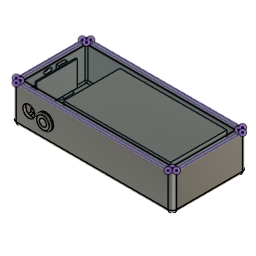
battery_box v25 (Autodesk Fusion 360 design; units mm, degrees)
Autodesk Fusion 360 part; units mm, degrees
sketch "Sketch1" plane through (0, 0, 0) normal (0, 0, 1) x (1, 0, 0) in component "box"
  line L0 (0, 0) -> (114, 0)
  line L1 (114, 0) -> (114, 53)
  line L2 (114, 53) -> (0, 53)
  line L3 (0, 53) -> (0, 0)
  dimension "d5" = 114
  dimension "d6" = 53
  constraint horizontal L0
  constraint vertical L1
  constraint horizontal L2
  constraint vertical L3
  constraint coincident L0.start L3.end
  measures "d5" distance of L0.start L0.end
  measures "d6" distance of L0.start L2.end
extrude "Extrude1" add sketch "Sketch1" along normal blind 30 makes body 1 in component "box"
fillet "Fillet1" radius 3 4 edges at (0, 0, 15) (0, 53, 15) (114, 53, 15) (114, 0, 15) on bodies 1 in component "box"
fillet "Fillet1" radius 3 2 faces at (38, 35.3333, 30) (38, 35.3333, 0) on bodies 1 in component "box"
shell "Shell1" thickness 2 removed faces 0 bodies 1 in component "box"
ref_plane "WorkPlane2" through (57, 26.5, 27) normal (0, 0, 1) x (1, 0, 0) in component "box"
split "Split1" by plane through (57, 26.5, 27) normal (0, 0, 1) bodies 1 makes body 2 at (39, 34.3333, 30) in component "box"
move_body "Move1" bodies 2 to x (1, 0, 0) y (0, 1, 0) z (0, 0, 1) at (88, 0, 0) in component "box"
sketch "Sketch5" plane through (0, 0, 27) normal (0, 0, 1) x (-1, 0, 0) in component "box"
  line L0 (-170, -3) -> (-170, -47)
  arc A0 (-90, -3) -> (-91, -2) centre (-91, -3) ccw
  line L1 (-91, -2) -> (-199, -2)
  arc A1 (-199, -2) -> (-200, -3) centre (-199, -3) ccw
  line L2 (-200, -3) -> (-200, -50)
  arc A2 (-200, -50) -> (-199, -51) centre (-199, -50) ccw
  line L3 (-199, -51) -> (-91, -51)
  arc A3 (-91, -51) -> (-90, -50) centre (-91, -50) ccw
  line L4 (-90, -50) -> (-90, -3)
  arc A4 (-88, -3) -> (-91, 0) centre (-91, -3) ccw
  line L5 (-88, -3) -> (-88, -50)
  arc A5 (-91, -53) -> (-88, -50) centre (-91, -50) ccw
  line L6 (-91, -53) -> (-199, -53)
  arc A6 (-202, -50) -> (-199, -53) centre (-199, -50) ccw
  line L7 (-202, -50) -> (-202, -3)
  arc A7 (-199, 0) -> (-202, -3) centre (-199, -3) ccw
  line L8 (-199, 0) -> (-91, 0)
sketch "Sketch1 (2)" plane through (0, 0, 0) normal (0, 0, 1) x (-1, 0, 0) in component "batteryholder"
  line L0 (0, 0) -> (-76, 0)
  line L1 (-76, 0) -> (-76, -40)
  line L2 (-76, -40) -> (0, -40)
  line L3 (0, -40) -> (0, 0)
  dimension "d20" = 76
  dimension "d21" = 40
  constraint horizontal L0
  constraint vertical L1
  constraint horizontal L2
  constraint vertical L3
  constraint coincident L0.start L3.end
  measures "d20" distance of L0.start L0.end
  measures "d21" distance of L0.start L2.end
extrude "Extrude1'" add sketch "Sketch1 (2)" along normal blind 20 separate body makes body 3 in component "batteryholder"
sketch "Sketch1 (3)" plane through (0, 0, 0) normal (0, 0, 1) x (-1, 0, 0) in component "charger"
sketch "Sketch2" plane through (0, 0, 0) normal (0, 0, 1) x (1, 0, 0) in component "charger"
  line L0 (0, 0) -> (29, 0)
  line L1 (29, 0) -> (29, 18)
  line L2 (29, 18) -> (0, 18)
  line L3 (0, 18) -> (0, 0)
  dimension "d24" = 29
  dimension "d25" = 18
  constraint horizontal L0
  constraint vertical L1
  constraint horizontal L2
  constraint vertical L3
  constraint coincident L0.start L3.end
  measures "d24" distance of L0.start L0.end
  measures "d25" distance of L0.start L2.end
extrude "Extrude1''" add sketch "Sketch2" along normal blind 1 separate body makes body 4 in component "charger"
sketch "Sketch3" plane through (0, 0, 0) normal (1, 0, 0) x (0, 1, 0) in component "charger"
  line L0 (9, 3) -> (0, 3)
  line L1 (0, 0) -> (9, 0)
  line L2 (0, 3) -> (0, 0)
  line L3 (9, 0) -> (9, 3)
  line L4 (18, 0) -> (0, 0)
  line L5 (0, 0) -> (0, 1)
  line L6 (0, 1) -> (18, 1)
  line L7 (18, 1) -> (18, 0)
  dimension "d33" = 9
  dimension "d34" = 3
  constraint horizontal L1
  constraint vertical L3
  constraint horizontal L0
  constraint vertical L2
  constraint coincident L1.start L2.end
  measures "d33" distance of L1.end L1.start
  measures "d34" distance of L0.end L1.start
extrude "Extrude2" add sketch "Sketch3" along normal blind 7 separate body contours L0 L2 L3 L6 | L1 L2 L3 L4 L5 L6 makes body 5 in component "charger"
move_body "Move1'" bodies 5 to x (1, 0, 0) y (0, 1, 0) z (0, 0, 1) at (0, 4, -3) in component "charger"
fillet "Fillet1'" radius 1 4 edges at (3.5, 4, 0) (3.5, 4, -3) (3.5, 13, 0) (3.5, 13, -3) on bodies 5 in component "charger"
move_body "Align5" bodies 5 to x (1, 0, 0) y (0, 1, 0) z (0, 0, 1) at (0, 0.5, 2) in component "charger"
move_body "Align6" bodies 5 to x (1, 0, 0) y (0, 1, 0) z (0, 0, 1) at (0, 0, -2) in component "charger"
combine "Combine1" operation add target body 4 tool bodies 5 in component "charger"
sketch "Sketch1 (4)" plane through (0, 0, 0) normal (1, 0, 0) x (0, 1, 0) in component "inputjack"
  circle A0 centre (0, 0) radius 5
  dimension "d64" = 10
  measures "d64" diameter of A0
extrude "Extrude1'''" add sketch "Sketch1 (4)" along normal blind 4 separate body makes body 6 in component "inputjack"
sketch "Sketch2 (2)" plane through (4, 0, 0) normal (1, 0, 0) x (0, 1, 0) in component "inputjack"
  circle A0 centre (0, 0) radius 5
  circle A1 centre (0, 0) radius 4
  dimension "d67" = 8
  constraint coincident A0.centre A1.centre
  measures "d67" diameter of A1
extrude "Extrude2'" add sketch "Sketch2 (2)" along normal blind 8 contours A1 bodies 6 in component "inputjack"
sketch "Sketch3 (2)" plane through (12, 0, 0) normal (1, 0, 0) x (0, 1, 0) in component "inputjack"
  circle A0 centre (0, 0) radius 4
  line L0 (-2.7, 1) -> (-3, 1)
  line L1 (-3, 1) -> (-3, -1)
  line L2 (-3, -1) -> (-2.7, -1)
  line L3 (-2.7, -1) -> (-2.7, 1)
  line L4 (2.7, -1) -> (3, -1)
  line L5 (3, 1) -> (2.7, 1)
  line L6 (3, -1) -> (3, 1)
  line L7 (2.7, 1) -> (2.7, -1)
  line L8 (0, 0) -> (-3, 0) construction
  line L9 (0, 0) -> (3, 0) construction
  point P0 (-3, 0)
  point P1 (3, 0)
  point P2 (-3, 0)
  point P3 (3, 0)
  dimension "d70" = 0.3
  dimension "d71" = 2
  dimension "d72" = 0.3
  dimension "d76" = 3
  constraint horizontal L0
  constraint vertical L1
  constraint horizontal L2
  constraint vertical L3
  constraint horizontal L5
  constraint vertical L7
  constraint horizontal L4
  constraint vertical L6
  constraint midpoint L1 P2
  constraint midpoint P3 L6
  constraint coincident P2 P0
  constraint coincident P3 P1
  constraint coincident A0.centre L8.start
  constraint perpendicular L1 L8
  constraint perpendicular L6 L9
  constraint equal L8 L9
  constraint equal L3 L6
  measures "d70" distance of L0.start L0.end
  measures "d71" distance of L0.start L2.end
  measures "d72" distance of L5.end L5.start
  measures "d76" distance of A0.centre P2
extrude "Extrude3" add sketch "Sketch3 (2)" along normal blind 4 contours L4 L5 L6 L7 bodies 6 in component "inputjack"
extrude "Extrude4" add sketch "Sketch3 (2)" along normal blind 6 contours L0 L1 L2 L3 bodies 6 in component "inputjack"
fillet "Fillet1''" radius 1 4 edges at (16, 2.85, 1) (16, 2.85, -1) (18, -2.85, 1) (18, -2.85, -1) on bodies 6 in component "inputjack"
sketch "Sketch4" plane through (0, -3, 0) normal (0, -1, 0) x (1, 0, 0) in component "inputjack"
  arc A0 (17, -1) -> (17, 1) centre (17, 0) ccw
  line L0 (17, 1) -> (12, 1)
  line L1 (12, 1) -> (12, -1)
  line L2 (12, -1) -> (17, -1)
  circle A1 centre (17.1, 0.0025) radius 0.25
  dimension "d83" = 0.5
  measures "d83" diameter of A1
sketch "Sketch5 (2)" plane through (0, 2.7, 0) normal (0, -1, 0) x (1, 0, 0) in component "inputjack"
  arc A0 (15, -1) -> (15, 1) centre (15, 0) ccw
  line L0 (15, 1) -> (12, 1)
  line L1 (12, 1) -> (12, -1)
  line L2 (12, -1) -> (15, -1)
  circle A1 centre (15, 0.0025) radius 0.25
  dimension "d84" = 0.5
  measures "d84" diameter of A1
extrude "Extrude5" cut sketch "Sketch4" against normal blind 1 contours A1 bodies 6 in component "inputjack"
extrude "Extrude6" cut sketch "Sketch5 (2)" against normal blind 1 contours A1 bodies 6 in component "inputjack"
sketch "Sketch7" plane through (0, 0, 0) normal (0, -1, 0) x (1, 0, 0) in component "box"
  line L0 (0, 0) -> (12, 0)
  line L1 (12, 0) -> (12, 14)
  line L2 (12, 14) -> (0, 14)
  line L3 (0, 14) -> (0, 0)
  line L4 (3, 3) -> (111, 3)
  line L5 (111, 3) -> (111, 27)
  line L6 (111, 27) -> (3, 27)
  line L7 (3, 27) -> (3, 3)
  line L8 (3, 3) -> (3, 27)
  line L9 (3, 0) -> (3, 3)
  dimension "d150" = 14
  dimension "d151" = 24
  dimension "d152" = 3
  dimension "d153" = 12
  constraint horizontal L0
  constraint vertical L1
  constraint horizontal L2
  constraint vertical L3
  constraint coincident L0.start L3.end
  measures "d150" distance of L0 L2
  measures "d151" distance of L4.start L6.end
  measures "d152" distance of L4.start L9.start
  measures "d153" distance of L1.end L2.end
combine "Combine1'" operation cut target body 1 tool bodies 6 body 6 seen with x (0, 1, 0) y (0, 0, 1) z (1, 0, 0) at (12, -4, 14) keep tools in component "box"
copy_body "Body->Comp2" bodies 2 removing the originals makes body 7 in component "lid"
sketch "Sketch8" plane through (0, 0, 0) normal (0, 1, 0) x (-1, 0, 0) in component "box"
  line L0 (-3, 3) -> (-3, 27)
  line L1 (-3, 27) -> (-107, 27)
  line L2 (-107, 27) -> (-107, 3)
  line L3 (-107, 3) -> (-3, 3)
  line L4 (-110, 0) -> (0, 0)
  circle A0 centre (-24, 14) radius 2.5
  line L5 (-3, 3) -> (-111, 3)
  line L6 (-111, 3) -> (-111, 27)
  line L7 (-111, 27) -> (-3, 27)
  line L8 (-3, 27) -> (-3, 3)
  circle A1 centre (-12, 14) radius 4
  point P0 (-12, 14)
  dimension "d90" = 5
  dimension "d154" = 12
  constraint horizontal A0.centre P0
  measures "d90" diameter of A0
  measures "d154" horizontal distance of A0.centre P0
extrude "Extrude3'" cut sketch "Sketch8" along normal blind 3 contours A0 bodies 1 in component "box"
sketch "Sketch9" plane through (2, 0, 0) normal (1, 0, 0) x (0, 1, 0) in component "box"
  line L0 (3, 3) -> (50, 3)
  line L1 (50, 3) -> (50, 27)
  line L2 (50, 27) -> (3, 27)
  line L3 (3, 27) -> (3, 3)
  line L4 (11.4717, 10.7056) -> (18.4717, 10.7056)
  line L5 (18.4717, 10.7056) -> (18.4717, 17.7056)
  line L6 (18.4717, 17.7056) -> (11.4717, 17.7056)
  line L7 (11.4717, 17.7056) -> (11.4717, 23.2056)
  line L8 (11.4717, 23.2056) -> (40.4717, 23.2056)
  line L9 (40.4717, 23.2056) -> (40.4717, 5.2056)
  line L10 (40.4717, 5.2056) -> (11.4717, 5.2056)
  line L11 (11.4717, 5.2056) -> (11.4717, 10.7056)
  line L12 (18.4717, 18.7056) -> (18.4717, 17.7056)
  line L13 (18.4717, 17.7056) -> (11.4717, 17.7056)
  line L14 (11.4717, 17.7056) -> (11.4717, 18.7056)
  line L15 (11.4717, 18.7056) -> (18.4717, 18.7056)
  line L16 (11.4717, 17.7056) -> (18.4717, 17.7056)
  line L17 (18.4717, 17.7056) -> (18.4717, 10.7056)
  line L18 (18.4717, 10.7056) -> (11.4717, 10.7056)
  line L19 (11.4717, 10.7056) -> (11.4717, 17.7056)
  line L20 (18.4717, 10.7056) -> (18.4717, 9.7056)
  line L21 (18.4717, 9.7056) -> (11.4717, 9.7056)
  line L22 (11.4717, 9.7056) -> (11.4717, 10.7056)
  line L23 (11.4717, 10.7056) -> (18.4717, 10.7056)
  line L24 (29.4717, 17.7056) -> (29.4717, 10.7056)
  line L25 (29.4717, 23.2056) -> (35.4717, 23.2056)
  line L26 (35.4717, 23.2056) -> (35.4717, 5.2056)
  line L27 (35.4717, 5.2056) -> (29.4717, 5.2056)
  line L28 (29.4717, 5.2056) -> (29.4717, 23.2056)
  line L29 (11.4717, 23.2056) -> (18.4717, 23.2056)
  line L30 (18.4717, 23.2056) -> (18.4717, 25.2056)
  line L31 (18.4717, 25.2056) -> (11.4717, 25.2056)
  line L32 (11.4717, 25.2056) -> (11.4717, 23.2056)
  line L33 (11.4717, 5.2056) -> (11.4717, 3.2056)
  line L34 (18.4717, 5.2056) -> (11.4717, 5.2056)
  line L35 (18.4717, 3.2056) -> (18.4717, 5.2056)
  line L36 (11.4717, 3.2056) -> (18.4717, 3.2056)
  line L37 (36.4717, 25.2056) -> (29.4717, 25.2056)
  line L38 (36.4717, 23.2056) -> (36.4717, 25.2056)
  line L39 (29.4717, 23.2056) -> (36.4717, 23.2056)
  line L40 (29.4717, 25.2056) -> (29.4717, 23.2056)
  line L41 (29.4717, 3.2056) -> (36.4717, 3.2056)
  line L42 (29.4717, 5.2056) -> (29.4717, 3.2056)
  line L43 (36.4717, 3.2056) -> (36.4717, 5.2056)
  line L44 (36.4717, 5.2056) -> (29.4717, 5.2056)
  line L45 (23.4717, 17.9111) -> (23.4717, 10.7056)
  ellipse E0 centre (23.4717, 22.2056) end of major axis (20.4717, 22.2056) minor radius 1.5
  line L46 (26.4717, 22.2056) -> (20.4717, 22.2056) construction
  line L47 (23.4717, 23.7056) -> (23.4717, 20.7056) construction
  line L48 (11.4717, 22.2056) -> (40.4717, 22.2056) construction
  line L49 (23.4717, 17.9111) -> (23.4717, 22.2056) construction
  dimension "d93" = -11
  dimension "d94" = 6
  dimension "d95" = 18
  dimension "d96" = 7
  dimension "d97" = 2
  dimension "d98" = 7
  dimension "d99" = 2
  dimension "d100" = 7
  dimension "d101" = 2
  dimension "d102" = 7
  dimension "d103" = 2
  dimension "d122" = -5
  dimension "d123" = 6
  dimension "d124" = 3
  dimension "d125" = 1
  constraint horizontal L25
  constraint vertical L26
  constraint horizontal L27
  constraint vertical L28
  constraint midpoint L24 L28
  constraint horizontal L29
  constraint vertical L30
  constraint horizontal L31
  constraint vertical L32
  constraint coincident L7.end L8.start
  constraint horizontal L36
  constraint vertical L35
  constraint horizontal L34
  constraint vertical L33
  constraint horizontal L39
  constraint vertical L38
  constraint horizontal L37
  constraint vertical L40
  constraint horizontal L41
  constraint vertical L43
  constraint horizontal L44
  constraint vertical L42
  constraint coincident E0 L46.start
  constraint coincident E0 L46.end
  constraint coincident E0 L47.start
  constraint coincident E0 L47.end
  constraint coincident L48 E0.centre
  constraint perpendicular L48 L49
  measures "d94" distance of L25.start L25.end
  measures "d95" distance of L25.start L27.end
  measures "d96" distance of L7.end L29.end
  measures "d97" distance of L7.end L31.end
  measures "d98" distance of L33.end L35.start
  measures "d99" distance of L33.end L10.end
  measures "d100" distance of L25.start L38.start
  measures "d101" distance of L25.start L37.end
  measures "d102" distance of L41.start L41.end
  measures "d103" distance of L27.end L41.start
  measures "d123" distance of E0
  measures "d124" distance of E0
extrude "Extrude4'" add sketch "Sketch9" along normal blind 6 contours L10 L33 L34 L35 L36 | L10 L27 L41 L42 L43 L44 bodies 1 in component "box"
chamfer "Chamfer1" distance 2 angle 45 2 edges at (8, 32.9717, 3.2056) (8, 14.9717, 3.2056) on bodies 1 in component "box"
extrude "Extrude5'" add sketch "Sketch9" along normal blind 1.9 separate body contours L8 L10 L24 L25 L26 L27 L28 L39 L44 makes body 8 in component "box"
sketch "Sketch10" plane through (0, 2, 0) normal (0, 1, 0) x (-1, 0, 0) in component "box"
  line L0 (-111, 3) -> (-3, 3)
  line L1 (-3, 3) -> (-3, 27)
  line L2 (-3, 27) -> (-111, 27)
  line L3 (-111, 27) -> (-111, 3)
  circle A0 centre (-12, 14) radius 4.25
  circle A1 centre (-24, 14) radius 2.5
  circle A2 centre (-12, 14) radius 4
  dimension "d112" = 8.5
  constraint coincident A0.centre A2.centre
  measures "d112" diameter of A0
extrude "Extrude6'" cut sketch "Sketch10" against normal blind 3.5 contours A0 | A2 bodies 1 in component "box"
sketch "Sketch11" plane through (0, 0, 0) normal (0, -1, 0) x (1, 0, 0) in component "box"
  line L0 (3, 27) -> (3, 3)
  line L1 (3, 3) -> (107, 3)
  line L2 (107, 3) -> (107, 27)
  line L3 (107, 27) -> (3, 27)
  circle A0 centre (12, 16) radius 2.5
  circle A1 centre (24, 14) radius 2.5
  line L4 (3, 3) -> (111, 3)
  line L5 (111, 3) -> (111, 27)
  line L6 (111, 27) -> (3, 27)
  line L7 (3, 27) -> (3, 3)
  circle A2 centre (24, 14) radius 5.5
  circle A3 centre (12, 14) radius 4.25
  dimension "d128" = 3
extrude "Extrude7" add sketch "Sketch11" along normal blind 2 contours A2 bodies 1 in component "box"
fillet "Fillet2" radius 1 1 edges at (18.8722, -2, 12.0111) on bodies 1 in component "box"
ref_plane "WorkPlane6" through (57, 1, 15) normal (0, -1, 0) x (1, 0, 0) in component "box"
mirror "Mirror1" about plane through (57, 1, 15) normal (0, -1, 0) of "Extrude7", "Fillet2" in component "box"
extrude "Extrude8" cut sketch "Sketch9" against normal blind 7 contours L8 E0 | L8 E0 bodies 1 in component "box"
sketch "Sketch1 (5)" plane through (0, 0, 27) normal (0, 0, -1) x (1, 0, 0) in component "lid"
  arc A0 (91, -2) -> (90, -3) centre (91, -3) ccw
  line L0 (91, -2) -> (199, -2)
  arc A1 (200, -3) -> (199, -2) centre (199, -3) ccw
  line L1 (200, -3) -> (200, -50)
  arc A2 (199, -51) -> (200, -50) centre (199, -50) ccw
  line L2 (199, -51) -> (91, -51)
  arc A3 (90, -50) -> (91, -51) centre (91, -50) ccw
  line L3 (90, -50) -> (90, -3)
  arc A4 (91, 0) -> (88, -3) centre (91, -3) ccw
  line L4 (88, -3) -> (88, -50)
  arc A5 (88, -50) -> (91, -53) centre (91, -50) ccw
  line L5 (91, -53) -> (199, -53)
  arc A6 (199, -53) -> (202, -50) centre (199, -50) ccw
  line L6 (202, -50) -> (202, -3)
  arc A7 (202, -3) -> (199, 0) centre (199, -3) ccw
  line L7 (199, 0) -> (91, 0)
  line L8 (92, -4) -> (198, -4)
  line L9 (92, -49) -> (92, -4)
  line L10 (198, -49) -> (92, -49)
  line L11 (198, -4) -> (198, -49)
  arc A8 (199.7, -3) -> (199, -2.3) centre (199, -3) ccw
  line L12 (91, -2.3) -> (199, -2.3)
  arc A9 (91, -2.3) -> (90.3, -3) centre (91, -3) ccw
  line L13 (90.3, -50) -> (90.3, -3)
  arc A10 (90.3, -50) -> (91, -50.7) centre (91, -50) ccw
  line L14 (199, -50.7) -> (91, -50.7)
  arc A11 (199, -50.7) -> (199.7, -50) centre (199, -50) ccw
  line L15 (199.7, -3) -> (199.7, -50)
  dimension "d134" = 2
  dimension "d137" = 0.3
sketch "Sketch13" plane through (0, 0, 27) normal (0, 0, 1) x (-1, 0, 0) in component "box"
  arc A0 (0, -3) -> (-3, 0) centre (-3, -3) ccw
  line L0 (-3, 0) -> (-111, 0)
  arc A1 (-111, 0) -> (-114, -3) centre (-111, -3) ccw
  line L1 (-114, -3) -> (-114, -50)
  arc A2 (-114, -50) -> (-111, -53) centre (-111, -50) ccw
  line L2 (-111, -53) -> (-3, -53)
  arc A3 (-3, -53) -> (0, -50) centre (-3, -50) ccw
  line L3 (0, -50) -> (0, -3)
  arc A4 (-2, -3) -> (-3, -2) centre (-3, -3) ccw
  line L4 (-2, -3) -> (-2, -50)
  arc A5 (-3, -51) -> (-2, -50) centre (-3, -50) ccw
  line L5 (-3, -51) -> (-111, -51)
  arc A6 (-112, -50) -> (-111, -51) centre (-111, -50) ccw
  line L6 (-112, -50) -> (-112, -3)
  arc A7 (-111, -2) -> (-112, -3) centre (-111, -3) ccw
  line L7 (-111, -2) -> (-3, -2)
  line L8 (-10.8727, -41.3772) -> (-23.8727, -41.3772)
  line L9 (-23.8727, -41.3772) -> (-23.8727, -22.1772)
  line L10 (-23.8727, -22.1772) -> (-10.8727, -22.1772)
  line L11 (-10.8727, -22.1772) -> (-10.8727, -41.3772)
  dimension "d132" = 13
  dimension "d133" = 19.2
  constraint horizontal L8
  constraint vertical L9
  constraint horizontal L10
  constraint vertical L11
  measures "d132" distance of L8.start L8.end
  measures "d133" distance of L8.start L10.end
extrude "Extrude1''''" add sketch "Sketch1 (5)" along normal blind 5 separate body contours A8 L12 A9 L13 A10 L14 A11 L15 makes body 9 in component "lid"
extrude "Extrude2''" add sketch "Sketch1 (5)" against normal blind 2.5 contours A0 L0 A1 L1 A2 L2 A3 L3 | A8 L12 A9 L13 A10 L14 A11 L15 bodies 7 9 in component "lid"
fillet "Fillet1'''" radius 0.28 8 edges at (90.505, 50.495, 27) (90.3, 26.5, 27) (90.505, 2.505, 27) (145, 2.3, 27) (199.495, 2.505, 27) (199.7, 26.5, 27) (199.495, 50.495, 27) (145, 50.7, 27) on bodies 7 in component "lid"
sketch "Sketch15" plane through (0, 2, 0) normal (0, 1, 0) x (-1, 0, 0) in component "box"
  circle A0 centre (-24, 14) radius 5.5
  line L0 (-111, 3) -> (-3, 3)
  line L1 (-3, 3) -> (-3, 27)
  line L2 (-3, 27) -> (-111, 27)
  line L3 (-111, 27) -> (-111, 3)
  line L4 (-111, 27) -> (-91, 27)
  line L5 (-3, 27) -> (-23, 27)
  line L6 (-4, 22) -> (-110, 22)
  circle A1 centre (-12, 14) radius 4.25
  line L7 (-31, 22) -> (-15, 22)
  line L8 (-15, 22) -> (-15, 25)
  line L9 (-15, 25) -> (-31, 25)
  line L10 (-31, 25) -> (-31, 22)
  point P0 (-111, 27)
  point P1 (-57, 27)
  point P2 (-57, 22)
  point P3 (-91, 22)
  point P4 (-23, 22)
  point P5 (-23, 22)
  dimension "d146" = 20
  dimension "d147" = 20
  dimension "d148" = 68
  dimension "d149" = 34
  dimension "d155" = 16
  dimension "d156" = 3
  dimension "d157" = 68
  dimension "d158" = 34
  constraint coincident P0 L2.end
  constraint horizontal L4
  constraint horizontal L5
  constraint coincident L1.end L2.start
  constraint coincident L2 P1
  constraint horizontal L7
  constraint vertical L8
  constraint horizontal L9
  constraint vertical L10
  constraint coincident L7 P5
  constraint midpoint L7 P5
  constraint vertical L5.end P5
  constraint vertical P1 P2
  constraint coincident P5 P4
  measures "d146" distance of P0 L4.end
  measures "d147" distance of L1.end L5.end
  measures "d148" distance of L4.end L5.end
  measures "d149" distance of L4.end P1
  measures "d155" distance of L7.start L7.end
  measures "d156" distance of L7.start L9.end
  measures "d157" distance of P3 P5
  measures "d158" distance of P2 P3
sketch "Sketch2 (3)" plane through (0, 0, 27) normal (0, 0, 1) x (-1, 0, 0)
  arc A0 (0, -3) -> (-3, 0) centre (-3, -3) ccw
  line L0 (-3, 0) -> (-111, 0)
  arc A1 (-111, 0) -> (-114, -3) centre (-111, -3) ccw
  line L1 (-114, -3) -> (-114, -50)
  arc A2 (-114, -50) -> (-111, -53) centre (-111, -50) ccw
  line L2 (-111, -53) -> (-3, -53)
  arc A3 (-3, -53) -> (0, -50) centre (-3, -50) ccw
  line L3 (0, -50) -> (0, -3)
  arc A4 (-2, -3) -> (-3, -2) centre (-3, -3) ccw
  line L4 (-2, -3) -> (-2, -50)
  arc A5 (-3, -51) -> (-2, -50) centre (-3, -50) ccw
  line L5 (-3, -51) -> (-111, -51)
  arc A6 (-112, -50) -> (-111, -51) centre (-111, -50) ccw
  line L6 (-112, -50) -> (-112, -3)
  arc A7 (-111, -2) -> (-112, -3) centre (-111, -3) ccw
  line L7 (-111, -2) -> (-3, -2)
  line L8 (-110, -49) -> (-110, -4)
  line L9 (-4, -49) -> (-110, -49)
  line L10 (-4, -4) -> (-4, -49)
  line L11 (-110, -4) -> (-4, -4)
  dimension "d159" = 2
extrude "Extrude2'''" [rolled back] along distance -6 taper angle 0
pasted_body "CutPasteBodies3" makes body 10 in component "box"
sketch "Sketch16" plane through (0, 0, 27) normal (0, 0, 1) x (-1, 0, 0) in component "box"
component "box" placed x (1, 0, 0) y (0, 1, 0) z (0, 0, 1) at (0, 0, 0)
component "batteryholder" placed x (1, 0, 0) y (0, 1, 0) z (0, 0, 1) at (29.8974, 6.9189, 6)
component "charger" placed x (0, 1, 0) y (0, 0, 1) z (1, 0, 0) at (5, 11.4717, 5.2056)
component "inputjack" placed x (0, 1, 0) y (0, 0, 1) z (1, 0, 0) at (12, -4, 14)
component "outputwire" placed x (1, 0, 0) y (0, 1, 0) z (0, 0, 1) at (0, 0, 0)
component "lid" placed x (1, 0, 0) y (0, 1, 0) z (0, 0, 1) at (-88, 0, 0) in component "box"
equation "d149 = d148 / 2"
equation "d150 = d151 / 2 + d152 - 1 mm"
equation "d158 = d148 / 2"
